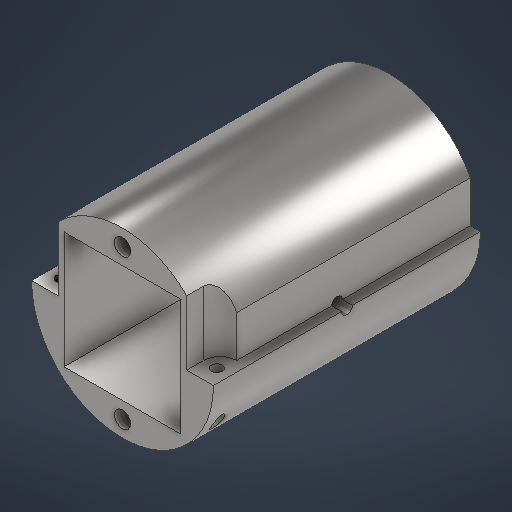
# Autodesk Inventor part: Part3_A_Y
Saved by Autodesk Inventor 2026 (Build 300175050, 175E)
## iProperties
Created: 2026-01-08
Part Number: Part3_A_Y
Material: 鋼、軟鋼
Document SubType Name: Modeling
Designer: Kota-Inoue
Density: 7.85 g/cm^3
Appearance: 半つや出し
Mass: 641.479 g
Surface Area: 319.402 cm^2
Volume: 81.7171 cm^3
Author: Kota-Inoue
Autodesk Inventor part; units mm, degrees
ref_plane "YZ Plane" through (0, 0, 0) normal (1, 0, 0) x (0, 1, 0)
ref_plane "XZ Plane" through (0, 0, 0) normal (0, 1, 0) x (-1, 0, 0)
ref_plane "XY Plane" through (0, 0, 0) normal (0, 0, 1) x (1, 0, 0)
sketch "スケッチ1" plane through (0, 0, 0) normal (0, 0, 1) x (1, 0, 0)
  circle A0 centre (0, 0) radius 27.25
  line L0 (17.5, 17.5) -> (-17.5, 17.5)
  line L1 (-17.5, 17.5) -> (-17.5, -17.5)
  line L2 (-17.5, -17.5) -> (17.5, -17.5)
  line L3 (17.5, -17.5) -> (17.5, 17.5)
  line L4 (17.5, 17.5) -> (-17.5, -17.5) construction
  line L5 (-17.5, 17.5) -> (17.5, -17.5) construction
  dimension "d0" = 54.5
  dimension "d6" = 35
  constraints: 12 end point, 2 midpoint, 2 parallel, 2 perpendicular, 1 centre point, 1 coincident, 1 horizontal
  measures "d0" diameter of A0
  measures "d6" distance of L0.start L0.end
extrude "押し出し1" add sketch "スケッチ1" against normal blind 80
sketch "スケッチ2" plane through (0, 0, 0) normal (0, 0, 1) x (1, 0, 0)
  line L0 (0, 42.4511) -> (0, -37.5489)
  line L1 (38.0038, 0) -> (-41.9962, 0)
  line L2 (27.25, 42.0143) -> (27.25, -37.9857)
  circle A0 centre (0, 0) radius 27.25 projected
  line L3 (17.5, 17.5) -> (17.5, -17.5) projected
  line L4 (19.25, 25) -> (27.25, 25)
  line L5 (27.25, 25) -> (27.25, -25)
  line L6 (27.25, -25) -> (19.25, -25)
  line L7 (19.25, -25) -> (19.25, 25)
  line L8 (19.25, 25) -> (27.25, -25) construction
  line L9 (27.25, 25) -> (19.25, -25) construction
  point P0 (17.5, 0)
  point P1 (23.25, 0)
  point P2 (19.25, 0)
  point P3 (27.25, 0)
  dimension "d13" = 9.75
  dimension "d14" = 8
  dimension "d15" = 50
  dimension "d19" = 54.5
  dimension "d103" = 1.75
  constraints: 18 end point, 3 midpoint, 3 point on line, 2 horizontal, 2 parallel, 2 vertical, 1 collinear, 1 perpendicular, 1 tangent
  measures "d13" distance from line of L2 point (17.5, 0)
  measures "d14" distance of L5.end L6.end
  measures "d15" distance of L4.end L5.end
  measures "d19" diameter of A0
  measures "d103" distance between parallel lines of L7 L3
extrude "押し出し2" cut sketch "スケッチ2" against normal blind 10 contours L7 L4 L2 A0 | A0 L1 L7 picked at (20.3822, 11.481)
sketch "スケッチ4" plane through (19.25, 0, 0) normal (0, 1, 0) x (1, 0, 0)
  line L0 (8, 0) -> (0, 0) projected
  line L1 (8, 0) -> (8, 10) projected
  line L2 (8, 10) -> (0, 10) projected
  line L3 (0, 0) -> (0, 10) projected
  line L4 (4, 10) -> (4, 0)
  line L5 (0, 5) -> (8, 5)
  point P0 (-19.25, 0)
  point P1 (4, 5)
  constraints: 6 midpoint, 4 end point
hole "穴1" at (23.25, 0, -5) direction (0, -1, 0) diameter 3.242 end through all thread size "M4x0.7" class "6H" standard "ISO Metric profile"
mirror "ミラー1" about plane through (0, 0, 0) normal (1, 0, 0) of "押し出し2", "穴1"
ref_plane "作業平面1" through (0, 0, -40) normal (0, 0, 1) x (1, 0, 0)
ref_plane "作業平面2" through (0, -17.5, 0) normal (1, 0, 0) x (0, 0, -1)
sketch "スケッチ6" plane through (0, 0, -80) normal (0, 0, -1) x (-1, 0, 0)
  circle A0 centre (0, 0) radius 27.25 projected
  circle A1 centre (0, 0) radius 22.375
  line L0 (0, 27.25) -> (0, -27.25)
  point P0 (0, 22.375)
  point P1 (0, -22.375)
  dimension "d45" = 44.75
  constraints: 4 point on circle, 2 end point, 2 point on line, 1 centre point, 1 midpoint, 1 vertical
  measures "d45" diameter of A1
hole "穴3" at (0, 22.375, -80) at (0, -22.375, -80) direction (0, 0, 1) diameter 4.917 depth 40 tip angle 118 thread size "M6x1" class "6H" standard "ISO Metric profile"
fillet "フィレット1" radius 5 2 edges at (19.25, 9.6437, -10) (-19.25, 9.6437, -10)
sketch "スケッチ8" plane through (0, 0, 0) normal (0, 0, 1) x (1, 0, 0)
  circle A0 centre (0, -22.375) radius 2.4585 projected
  circle A1 centre (0, 22.375) radius 2.4585 projected
  circle A2 centre (0, 0) radius 27.25 projected
  line L0 (17.5, -17.5) -> (17.5, 17.5) projected
  line L1 (17.5, 17.5) -> (-17.5, 17.5) projected
  line L2 (-17.5, 17.5) -> (-17.5, -17.5) projected
  line L3 (-17.5, -17.5) -> (17.5, -17.5) projected
hole "穴5" at (0, 22.375, 0) at (0, -22.375, 0) direction (0, 0, -1) diameter 4.917 depth 40 tip angle 118 thread size "M6x1" class "6H" standard "ISO Metric profile"
sketch "スケッチ9" plane through (0, 0, 0) normal (0, 0, 1) x (1, 0, 0)
  circle A0 centre (0, -23.375) radius 2.4585
  circle A1 centre (0, 23.375) radius 2.4585
  circle A2 centre (0, 0) radius 27.25
  line L0 (0, 42.5051) -> (0, -37.4949)
  line L1 (38.0038, 0) -> (-41.9962, 0)
  circle A3 centre (0, 0) radius 22.375
  line L2 (-17.5, 17.5) -> (17.5, 17.5) projected
  line L3 (27.25, 30.7275) -> (27.25, -9.2725)
  line L4 (24.25, 0) -> (27.25, 0)
  line L5 (27.25, 0) -> (27.25, 13)
  line L6 (27.25, 13) -> (24.25, 13)
  line L7 (24.25, 13) -> (24.25, 0)
  line L8 (24.25, 0) -> (27.25, 13) construction
  line L9 (27.25, 0) -> (24.25, 13) construction
  point P0 (0, 0)
  point P1 (18.5, 0)
  point P2 (-47.5735, 26.9542)
  point P3 (-39.5735, 26.9542)
  point P4 (-39.5735, 51.9542)
  point P5 (0, 22.375)
  point P6 (0, -22.375)
  point P7 (0, 20.9165)
  point P8 (0, 17.5)
  point P9 (0, 17.5)
  point P10 (25.75, 6.5)
  point P11 (24.25, 0)
  dimension "d76" = 44.75
  dimension "d85" = 40
  dimension "d86" = 3
  dimension "d87" = 13
  dimension "d104" = 54.5
  constraints: 18 end point, 5 point on line, 4 midpoint, 3 centre point, 3 horizontal, 3 vertical, 2 parallel, 2 perpendicular, 2 point on circle, 1 tangent, 1 vertical alignment, 2 other
  measures "d76" diameter of A3
  measures "d85" distance of L3.start L3.end
  measures "d86" distance of L6.end L5.end
  measures "d87" distance of L4.end L5.end
  measures "d104" diameter of A2
extrude "押し出し4" cut sketch "スケッチ9" against normal blind 80 contours L7 A2 L1 | A2 L7 L6 L3
sketch "スケッチ10" plane through (24.25, 0, -10) normal (1, 0, 0) x (0, 0, -1)
  line L0 (70, -27.25) -> (70, 27.25) projected
  line L1 (-10, 0) -> (-10, -27.25) projected
  line L2 (-10, 0) -> (70, 0) projected
  line L3 (0, 12.4298) -> (70, 12.4298) projected
  line L4 (-18.5995, 0) -> (81.4005, 0)
  line L5 (30, 31.8936) -> (30, -34.2066)
  line L6 (-10, 0) -> (30, 0)
  point P0 (30, 0)
  point P1 (30, 0)
  dimension "d90" = 80
  dimension "d91" = 12.4298
  dimension "d95" = 40
  constraints: 6 end point, 2 midpoint, 2 point on line, 1 horizontal, 1 perpendicular
  measures "d90" distance between parallel lines of L0 L1
  measures "d91" distance between parallel lines of L2 L3
  measures "d95" distance of point (30, 0) L1.start
hole "穴6" at (24.25, 0, -40) direction (-1, 0, 0) diameter 3.242 depth 7 tip angle 118 start extended yes thread size "M4x0.7" class "6H" standard "ISO Metric profile"
mirror "ミラー3" about plane through (0, 0, 0) normal (1, 0, 0) of "穴6"
mirror "ミラー4" about plane through (0, 0, 0) normal (1, 0, 0) of "押し出し4"
sketch "スケッチ11" plane through (0, 0, -40) normal (0, 0, 1) x (1, 0, 0)
  point P0 (0, 0)
